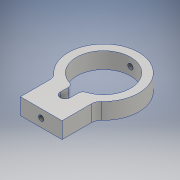
# Autodesk Inventor part: LaserTubeClamp
Saved by Autodesk Inventor 2017 SP1 (Build 210196100, 196)
## iProperties
Created: 2015-08-04
Part Number: LaserTubeClamp
Material: Generic
Document SubType Name: Modeling
Designer: Conor Mow-Lowry
Density: 1 g/cm^3
Appearance: Aluminum - Flat
Author: Conor Mow-Lowry
Autodesk Inventor part; units mm, degrees
ref_plane "YZ Plane" through (0, 0, 0) normal (1, 0, 0) x (0, 1, 0)
sketch "Sketch1" plane through (0, 0, 0) normal (0, 0, 1) x (1, 0, 0)
  circle A0 centre (0, 0) radius 15 construction
  circle A1 centre (0, 0) radius 16.5
  circle A2 centre (0, 0) radius 21.5
  line L0 (0, 0) -> (26.2932, 0) construction
  line L1 (0, 0) -> (0, -21.5) construction
  line L2 (-12.7, -38.1) -> (12.7, -38.1)
  line L3 (12.7, -38.1) -> (12.7, -17.3482)
  line L4 (12.7, -17.3482) -> (-12.7, -17.3482)
  line L5 (-12.7, -17.3482) -> (-12.7, -38.1)
  line L6 (-12.7, -38.1) -> (12.7, -17.3482) construction
  line L7 (12.7, -38.1) -> (-12.7, -17.3482) construction
  point P0 (0, -27.7241)
  point P1 (0, -27.7241)
  dimension "d0" = 30
  dimension "d1" = 33
  dimension "d2" = 43
  dimension "d7" = 25.4
  dimension "d8" = 38.1
  constraints: 16 end point, 3 centre point, 3 coincident, 3 midpoint, 2 horizontal, 2 parallel, 2 point on circle, 1 perpendicular, 1 point on line, 1 vertical
  measures "d0" diameter of A0
  measures "d1" diameter of A1
  measures "d2" diameter of A2
  measures "d7" distance of L3.end L4.end
  measures "d8" distance between parallel lines of L2 L0
extrude "Extrusion1" add sketch "Sketch1" along normal blind 10
fillet "Fillet2" radius 6 2 edges at (12.7, -17.3482, 5) (-12.7, -17.3482, 5)
sketch "Sketch3" plane through (-12.7, -38.1, 0) normal (0, -1, 0) x (1, 0, 0)
  line L0 (0, 0) -> (0, 10) projected
  line L1 (12.7, 0) -> (12.7, 10) construction
  line L2 (-3.8, 10) -> (29.2, 10) construction
  line L3 (0, 5) -> (25.4, 5) construction
  line L4 (25.4, 10) -> (25.4, 0) construction
  point P0 (0.8561, 10)
  point P1 (24.5439, 10)
  point P2 (12.7, 5)
  constraints: 4 end point, 4 midpoint
hole "Hole1" at (0, -38.1, 5) direction (0, 1, 0) diameter 3.242 depth 10 tip angle 118 thread size "M4x0.7" class "6H" standard "ANSI Metric M Profile"
ref_plane "Work Plane1" through (0, 21.5, 0) normal (0, 1, 0) x (-1, 0, 0)
sketch "Sketch4" plane through (0, 21.5, 0) normal (0, 1, 0) x (-1, 0, 0)
  line L0 (0, 0) -> (0, 10) construction
  line L1 (12.7, 10) -> (-12.7, 10) construction
  circle A0 centre (0, 5) radius 1.621 construction
  point P0 (0, 5)
  constraints: 2 end point, 1 coincident, 1 midpoint
hole "Hole2" at (0, 21.5, 5) direction (0, -1, 0) diameter 3.302 depth 12.3 tip angle 118 thread size "8-32 UNC" class "2B" standard "ANSI Unified Screw Threads"
sketch "Sketch5" plane through (0, 0, 10) normal (0, 0, 1) x (1, 0, 0)
  circle A0 centre (0, 0) radius 16.5 projected
  arc A1 (14.62, -15.7641) -> (-14.62, -15.7641) centre (0, 0) ccw projected
  line L0 (0, 0) -> (0, -38.1) construction
  line L1 (1.621, -38.1) -> (-1.621, -38.1) construction
  circle A2 centre (0, -23.5) radius 3
  line L2 (-3, -23.5) -> (-3, -16.225)
  line L3 (3, -23.5) -> (3, -16.225)
  line L4 (-12.7, -20.1633) -> (-12.7, -38.1) projected
  line L5 (12.7, -38.1) -> (12.7, -20.1633) projected
  line L6 (-12.7, -26.5) -> (12.7, -26.5) construction
  line L7 (12.7, -38.1) -> (12.7, -20.1633) construction
  line L8 (-10.4966, -16.5) -> (9.259, -16.5) construction
  dimension "d28" = 6
  dimension "d32" = 10
  constraints: 10 end point, 4 point on circle, 4 tangent, 3 point on line, 2 vertical, 1 centre point, 1 horizontal, 1 midpoint, 1 perpendicular
  measures "d28" diameter of A2
  measures "d32" distance between parallel lines of L6 L8
extrude "Extrusion3" cut sketch "Sketch5" against normal through all contours A0 L3 A2 L2 | A2
fillet "Fillet4" radius 3 2 edges at (-3, -16.225, 5) (3, -16.225, 5)
ref_plane "Work Plane2" through (0, 0, 5) normal (0, 0, 1) x (1, 0, 0)
body "Solid1"
